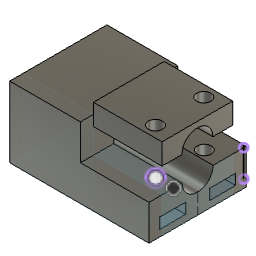
kryt_vystup v4 (Autodesk Fusion 360 design; units mm, degrees)
Autodesk Fusion 360 part; units mm, degrees
sketch "Sketch2" plane through (0, 0, 0) normal (0, 0, 1) x (1, 0, 0) in component "Component"
  line L0 (0, 0) -> (16, 0)
  line L1 (16, 0) -> (16, 16)
  line L2 (16, 16) -> (0, 16)
  line L3 (0, 16) -> (0, 0)
  dimension "d9" = 16
  dimension "d10" = 16
  constraint horizontal L0
  constraint vertical L1
  constraint horizontal L2
  constraint vertical L3
  constraint coincident L0.start L3.end
  measures "d9" distance of L0.start L0.end
  measures "d10" distance of L0.start L2.end
extrude "Extrude2" add sketch "Sketch2" along normal blind 16 makes body 1 in component "Component"
sketch "Sketch3" plane through (0, 0, 0) normal (0, -1, 0) x (1, 0, 0) in component "Component"
  line L0 (0, 0) -> (16, 0)
  line L1 (16, 0) -> (16, 16)
  line L2 (16, 16) -> (0, 16)
  line L3 (0, 16) -> (0, 0)
sketch "Sketch4" plane through (16, 0, 0) normal (1, 0, 0) x (0, 1, 0) in component "Component"
  line L0 (0, 0) -> (16, 0)
  line L1 (16, 0) -> (16, 16)
  line L2 (16, 16) -> (0, 16)
  line L3 (0, 16) -> (0, 0)
  line L4 (0, 8) -> (16, 8) construction
  line L5 (8, 16) -> (8, 0) construction
  circle A0 centre (8, 8) radius 3.5
  line L6 (4.5, 8) -> (0, 8)
  line L7 (8, 4.5) -> (0, 4.5)
  line L8 (0, 8) -> (0, 4.5)
  line L9 (16, 8) -> (0, 8) construction
  line L10 (16, 8) -> (16, 4.5)
  line L11 (8, 4.5) -> (16, 4.5)
  line L12 (4.5, 8) -> (0, 8)
  line L13 (0, 8) -> (0, 11.25)
  line L14 (8, 11.5) -> (0, 11.5)
  line L15 (8, 11.5) -> (16, 11.5)
  line L16 (16, 8) -> (16, 11.5)
  line L17 (11.5, 8) -> (16, 8)
  line L18 (0, 0) -> (16, 0)
  line L19 (16, 0) -> (16, 4.5)
  line L20 (0, 11.25) -> (0, 12.75)
  line L21 (16, 11.25) -> (16, 12.75)
  line L22 (0, 12.75) -> (16, 12.75)
  dimension "d15" = 7
  dimension "d51" = 3.5
  dimension "d52" = 1.5
  constraint midpoint L3 L4.start
  constraint midpoint L1 L4.end
  constraint midpoint L2 L5.start
  constraint midpoint L0 L5.end
  constraint midpoint L4 A0.centre
  constraint coincident L4 L6.start
  constraint coincident A0 L6.start
  constraint coincident L5 L7.start
  constraint coincident A0 L7.start
  constraint coincident L3 L7.end
  constraint tangent A0 L7
  constraint symmetric L4.start L5 L4.end
  constraint symmetric L4.end L5 L4.start
  constraint symmetric L5 L7.start L11.start
  constraint symmetric L5 L7.end L10.end
  constraint symmetric L4.start L9 L6.end
  constraint symmetric L6.start L9 L12.start
  constraint symmetric L7.start L9 L14.start
  constraint symmetric L7.end L9 L14.end
  constraint symmetric L4.end L9 L10.start
  constraint symmetric L9 L10.end L15.end
  constraint symmetric L9 L7.start L14.start
  constraint coincident A0 L17.start
  constraint coincident L9 L17.start
  constraint coincident L0.start L3.end
  constraint coincident L0.end L1.start
  constraint perpendicular L14 L20
  constraint symmetric L5 L13.end L21.start
  constraint symmetric L5 L20.end L21.end
  measures "d15" diameter of A0
  measures "d51" distance of L4.start L14.end
  measures "d52" distance of L13.end L20.end
extrude "Extrude4" add sketch "Sketch4" along normal blind 15.5 separate body contours L3 A0 L6 L7 L8 L12 | L1 A0 L10 L11 L17 makes body 2 in component "Component"
extrude "Extrude9" add sketch "Sketch4" along normal blind 15.5 contours L0 L1 L3 L7 L11 L18 L19 bodies 1 2 in component "Component"
extrude "Extrude3" cut sketch "Sketch4" along normal mid plane 84 contours A0 bodies 1 in component "Component"
sketch "Sketch6" plane through (0, 0, 8) normal (0, 0, 1) x (-1, 0, 0) in component "Component"
  line L0 (-16, 0) -> (-31.5, 0)
  line L1 (-31.5, 0) -> (-31.5, -4.5)
  line L2 (-31.5, -4.5) -> (-16, -4.5)
  circle A0 centre (-27.5, -2.5) radius 1.6
  circle A1 centre (-27.5, -13.5) radius 1.6
  line L3 (-16, -4.5) -> (-16, 0)
  dimension "d20" = 3.2
  dimension "d21" = 3.2
  measures "d20" diameter of A0
  measures "d21" diameter of A1
extrude "Extrude5" cut sketch "Sketch6" against normal blind 6.5 contours A0 | A1 bodies 1 in component "Component"
extrude "Extrude1" add sketch "Sketch4" along normal blind 15.5 from surface at 1 separate body contours L3 A0 L6 L12 L13 L14 L20 | L1 A0 L15 L16 L17 L21 | L1 L3 L14 L15 L20 L21 L22 makes body 3 in component "Component'"
sketch "Sketch8" plane through (0, 0, 8) normal (0, 0, 1) x (-1, 0, 0) in component "Component"
  line L0 (-16, -4.5) -> (-16, 0)
  line L1 (-16, 0) -> (-31.5, 0)
  line L2 (-31.5, 0) -> (-31.5, -4.5)
  line L3 (-31.5, -4.5) -> (-16, -4.5)
  line L4 (-27.4987, -2.525) -> (-31.5, -2.525) construction
  circle A0 centre (-27.5, -2.5) radius 1.6
  constraint coincident L2 L4.end
  constraint perpendicular L2 L4
sketch "Sketch1" plane through (27.5314, 0, 0) normal (1, 0, 0) x (0, 1, 0)
  arc A0 (3.5271, 9.0328) -> (10.5271, 9.0328) centre (7.0271, 9.0328) ccw
  line L0 (3.5271, 9.0328) -> (-0.9729, 9.0328)
  line L1 (-0.9729, 9.0328) -> (-0.9729, 1.0328)
  line L2 (-0.9729, 1.0328) -> (15.0271, 1.0328)
  line L3 (15.0271, 1.0328) -> (15.0271, 9.0328)
  line L4 (15.0271, 9.0328) -> (10.5271, 9.0328)
  line L5 (7.0271, 5.5328) -> (7.0271, 1.0328) construction
  constraint midpoint A0 L5.start
  constraint midpoint L2 L5.end
move_face "OffsetFaces1" offset 3 1 faces at (5.3333, 0, 8) on bodies 1 in component "Component"
move_face "OffsetFaces2" offset 3 1 faces at (5.3333, 16, 8) on bodies 1 in component "Component"
sketch "Sketch9" plane through (31.5, 0, 0) normal (1, 0, 0) x (0, 1, 0) in component "Component"
  arc A0 (4.5, 8) -> (11.5, 8) centre (8, 8) ccw
  line L0 (4.5, 8) -> (-3, 8)
  line L1 (-3, 8) -> (-3, 0)
  line L2 (-3, 0) -> (19, 0)
  line L3 (19, 0) -> (19, 8)
  line L4 (19, 8) -> (11.5, 8)
  line L5 (13.4842, 1.5) -> (16.5842, 1.5)
  line L6 (13.4638, 1.5) -> (10.7138, 1.5)
  line L7 (10.7138, 1.5) -> (10.7138, 3.9)
  line L8 (10.7138, 3.9) -> (16.5842, 3.9)
  line L9 (16.5842, 3.9) -> (16.5842, 1.5)
  line L10 (8, 4.5) -> (8, 0)
  line L11 (5.2862, 1.5) -> (5.2862, 3.9)
  line L12 (2.5362, 1.5) -> (5.2862, 1.5)
  line L13 (2.5158, 1.5) -> (-0.5842, 1.5)
  line L14 (-0.5842, 3.9) -> (-0.5842, 1.5)
  line L15 (5.2862, 3.9) -> (-0.5842, 3.9)
  line L16 (13.4842, 1.5) -> (13.4638, 1.5)
  line L17 (2.5158, 1.5) -> (2.5362, 1.5)
  dimension "d44" = 3.1
  dimension "d45" = 2.4
  constraint perpendicular L6 L7
  constraint vertical L9
  constraint symmetric L5.start L10 L13.start
  constraint symmetric L5.end L10 L13.end
  constraint symmetric L6.start L10 L12.start
  constraint symmetric L6.end L10 L11.start
  constraint symmetric L7.end L10 L11.end
  constraint symmetric L8.end L10 L14.start
  constraint parallel L6 L16
  constraint parallel L12 L17
  measures "d44" distance of L5.start L5.end
  measures "d45" distance of L6.end L7.end
sketch "Sketch10" plane through (0, 0, 0) normal (0, 0, -1) x (1, 0, 0) in component "Component"
  line L0 (0, 3) -> (0, -19)
  line L1 (0, -19) -> (31.5, -19)
  line L2 (31.5, -19) -> (31.5, 3)
  line L3 (31.5, 3) -> (0, 3)
extrude "Extrude10" cut sketch "Sketch9" against normal blind 7.5 contours L11 L12 L13 L14 L15 L17 bodies 1 in component "Component"
sketch "Sketch11" plane through (31.5, 0, 0) normal (1, 0, 0) x (0, 1, 0) in component "Component"
  line L0 (5.2862, 3.9) -> (5.2862, 1.5)
  line L1 (5.2862, 1.5) -> (-0.5842, 1.5)
  line L2 (-0.5842, 1.5) -> (-0.5842, 3.9)
  line L3 (-0.5842, 3.9) -> (5.2862, 3.9)
  arc A0 (4.5, 8) -> (11.5, 8) centre (8, 8) ccw
  line L4 (4.5, 8) -> (-3, 8)
  line L5 (-3, 8) -> (-3, 0)
  line L6 (-3, 0) -> (19, 0)
  line L7 (19, 0) -> (19, 8)
  line L8 (19, 8) -> (11.5, 8)
  line L9 (8, 4.5) -> (8, 0) construction
  line L10 (8, 4.5) -> (8, 0)
  line L11 (16.5842, 1.5) -> (16.5842, 3.9)
  line L12 (10.7138, 1.5) -> (16.5842, 1.5)
  line L13 (10.7138, 3.9) -> (10.7138, 1.5)
  line L14 (16.5842, 3.9) -> (10.7138, 3.9)
  constraint midpoint A0 L9.start
  constraint midpoint L6 L9.end
  constraint symmetric L0.start L10 L13.start
  constraint symmetric L0.end L10 L12.start
  constraint symmetric L1.end L10 L11.start
  constraint symmetric L2.end L10 L11.end
extrude "Extrude11" cut sketch "Sketch11" against normal blind 7.5 contours L11 L12 L13 L14 bodies 1 in component "Component"
sketch "Sketch2 (2)" plane through (0, 0, 0) normal (0, 0, 1) x (1, 0, 0)
sketch "Sketch5" plane through (0.0964, 1.4364, 18.8896) normal (0, 0, 1) x (-1, 0, 0)
  line L0 (-16.82, -30.7145) -> (-16.82, -14.7145)
  line L1 (-16.82, -14.7145) -> (-32.32, -14.7145)
  line L2 (-32.32, -14.7145) -> (-32.32, -30.7145)
  line L3 (-32.32, -30.7145) -> (-16.82, -30.7145)
  line L4 (-32.32, -17.2395) -> (-28.3199, -17.2395) construction
  line L5 (-28.3199, -17.2395) -> (-28.3199, -19.4645) construction
  line L6 (-32.32, -22.7145) -> (-16.82, -22.7145) construction
  line L7 (-28.3199, -28.1895) -> (-28.3199, -25.9645) construction
  line L8 (-32.32, -28.1895) -> (-28.3199, -28.1895) construction
  circle A0 centre (-28.3199, -17.2395) radius 1.45
  circle A1 centre (-28.3199, -28.1895) radius 1.45
  point P0 (-28.3199, -28.1895)
  dimension "d53" = 4.0001
  dimension "d55" = 2.225
  dimension "d56" = 2.9
  constraint coincident L2 L4.start
  constraint perpendicular L2 L4
  constraint perpendicular L4 L5
  constraint midpoint L2 L6.start
  constraint midpoint L0 L6.end
  constraint symmetric L4.start L6 L8.start
  constraint symmetric L4.end L6 P0
  constraint symmetric L5.end L6 L7.end
  constraint coincident L4.end L5.start
  constraint symmetric L6 L4.end P0
  constraint symmetric L6 A0 A1
  measures "d53" distance of L4.start L4.end
  measures "d55" distance of L4.end L5.end
  measures "d56" diameter of A0
extrude "Extrude3'" cut sketch "Sketch5" against normal blind 6 contours A0 | A1 sketch seen with x (1, 0, 0) y (0, 1, 0) z (0, 0, 1) at (0.0836, -16.151, -6.1396) bodies 3 in component "Component'"
sketch "Sketch3 (2)" plane through (0, 0, 2.5328) normal (0, 0, 1) x (-1, 0, 0)
  line L0 (-27.5314, 1.5571) -> (-27.5314, -4.3133)
  line L1 (-27.5314, -4.3133) -> (-20.0314, -4.3133)
  line L2 (-20.0314, -4.3133) -> (-20.0314, 1.5571)
  line L3 (-20.0314, 1.5571) -> (-27.5314, 1.5571)
sketch "Sketch6 (2)" plane through (27.5314, 0, 0) normal (1, 0, 0) x (0, 1, 0)
  line L0 (9.7409, 2.5328) -> (9.7409, 4.9328)
  line L1 (9.7409, 4.9328) -> (15.6113, 4.9328)
  line L2 (15.6113, 4.9328) -> (15.6113, 2.5328)
  line L3 (15.6113, 2.5328) -> (9.7409, 2.5328)
  line L4 (4.3133, 4.9328) -> (4.3133, 2.5328)
  line L5 (4.3133, 2.5328) -> (-1.5571, 2.5328)
  line L6 (-1.5571, 2.5328) -> (-1.5571, 4.9328)
  line L7 (-1.5571, 4.9328) -> (4.3133, 4.9328)
  arc A0 (3.5271, 9.0328) -> (10.5271, 9.0328) centre (7.0271, 9.0328) ccw
  line L8 (3.5271, 9.0328) -> (-3.9729, 9.0328)
  line L9 (-3.9729, 9.0328) -> (-3.9729, 1.0328)
  line L10 (-3.9729, 1.0328) -> (18.0271, 1.0328)
  line L11 (18.0271, 1.0328) -> (18.0271, 9.0328)
  line L12 (18.0271, 9.0328) -> (10.5271, 9.0328)
sketch "Sketch7" plane through (0, 0, 18.8896) normal (0, 0, 1) x (-1, 0, 0)
  circle A0 centre (-28.4163, -18.676) radius 1.45
  circle A1 centre (-28.4163, -29.626) radius 1.45
  line L0 (-16.9164, -32.151) -> (-16.9164, -16.151)
  line L1 (-16.9164, -16.151) -> (-32.4164, -16.151)
  line L2 (-32.4164, -16.151) -> (-32.4164, -32.151)
  line L3 (-32.4164, -32.151) -> (-16.9164, -32.151)
  circle A2 centre (-28.4163, -18.676) radius 1.6
  circle A3 centre (-28.4163, -29.626) radius 1.6
  dimension "d59" = 3.2
  dimension "d60" = 3.2
  constraint concentric A0 A2
  constraint concentric A1 A3
  measures "d59" diameter of A2
  measures "d60" diameter of A3
extrude "Extrude12" cut sketch "Sketch7" against normal blind 16 contours A2 sketch seen with x (1, 0, 0) y (0, 1, 0) z (0, 0, 1) at (3.9686, 0.9729, -1.0328) bodies 1 in component "Component"
extrude "Extrude4'" cut sketch "Sketch7" against normal blind 16 contours A2 sketch seen with x (1, 0, 0) y (0, 1, 0) z (0, 0, 1) at (0.0836, -16.151, -6.1396) bodies 3 in component "Component'"
sketch "Sketch1 (2)" plane through (0, 0, 12.75) normal (0, 0, 1) x (-1, 0, 0) in component "Component'"
  circle A0 centre (-28.4999, -2.525) radius 1.6
  circle A1 centre (-28.4999, -13.475) radius 1.45
  line L0 (-17, -16) -> (-17, 0)
  line L1 (-17, 0) -> (-32.5, 0)
  line L2 (-32.5, 0) -> (-32.5, -16)
  line L3 (-32.5, -16) -> (-17, -16)
  circle A2 centre (-28.4999, -13.475) radius 1.6
  dimension "d65" = 3.2
  constraint concentric A1 A2
  measures "d65" diameter of A2
extrude "Extrude5'" cut sketch "Sketch1 (2)" against normal blind 13 contours A2 bodies 3 in component "Component'"
sketch "Sketch8 (2)" plane through (27.5314, 0, 0) normal (1, 0, 0) x (0, 1, 0)
  line L0 (17.5273, 2.8896) -> (17.3429, 2.8896)
  line L1 (17.3429, 9.0328) -> (10.5271, 9.0328)
  arc A0 (3.5271, 9.0328) -> (10.5271, 9.0328) centre (7.0271, 9.0328) ccw
  line L2 (3.5271, 9.0328) -> (-3.9729, 9.0328)
  line L3 (-3.9729, 9.0328) -> (-3.9729, 1.0328)
  line L4 (-3.9729, 1.0328) -> (18.0271, 1.0328)
  line L5 (18.0271, 1.0328) -> (18.0271, 9.0328)
  line L6 (18.0271, 9.0328) -> (17.5273, 9.0328)
  line L7 (4.3133, 4.9328) -> (4.3133, 2.5328)
  line L8 (4.3133, 2.5328) -> (-1.5571, 2.5328)
  line L9 (-1.5571, 2.5328) -> (-1.5571, 4.9328)
  line L10 (-1.5571, 4.9328) -> (4.3133, 4.9328)
  line L11 (9.7409, 2.5328) -> (9.7409, 4.9328)
  line L12 (9.7409, 4.9328) -> (15.6113, 4.9328)
  line L13 (15.6113, 4.9328) -> (15.6113, 2.5328)
  line L14 (15.6113, 2.5328) -> (9.7409, 2.5328)
component "Component" placed x (1, 0, 0) y (0, 1, 0) z (0, 0, 1) at (-3.9686, -0.9729, 1.0328)
component "Component'" placed x (1, 0, 0) y (0, 1, 0) z (0, 0, 1) at (-0.0836, 16.151, 6.1396)
